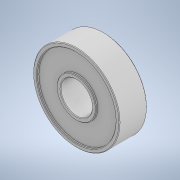
# Autodesk Inventor part: SS608-2RS
Saved by Autodesk Inventor 2021 (Build 250183000, 183)
## iProperties
Created: 2021-02-26
Part Number: SS608-2RS
Material: Generic
Document SubType Name: Modeling
Designer: Viktor
Density: 1 g/cm^3
Appearance: Default
Author: Viktor
Autodesk Inventor part; units mm, degrees
ref_plane "YZ Plane" through (0, 0, 0) normal (1, 0, 0) x (0, 1, 0)
ref_plane "XZ Plane" through (0, 0, 0) normal (0, 1, 0) x (-1, 0, 0)
ref_plane "XY Plane" through (0, 0, 0) normal (0, 0, 1) x (1, 0, 0)
sketch "Sketch1" plane through (0, 0, 0) normal (0, 0, 1) x (1, 0, 0)
  circle A0 centre (0, 0) radius 11
  circle A1 centre (0, 0) radius 4
  dimension "d0" = 22
  dimension "d1" = 8
  constraints: 2 centre point, 2 coincident
  measures "d0" diameter of A0
  measures "d1" diameter of A1
extrude "Extrusion1" add sketch "Sketch1" along normal mid plane 7
sketch "Sketch2" plane through (0, 0, 3.5) normal (0, 0, 1) x (1, 0, 0)
  circle A0 centre (0, 0) radius 10
  circle A1 centre (0, 0) radius 5
  circle A2 centre (0, 0) radius 11 projected
  circle A3 centre (0, 0) radius 4 projected
  dimension "d4" = 1
  dimension "d5" = 1
  constraints: 2 centre point, 2 coincident
  measures "d4" radial gap between concentric circles of A2 A0
  measures "d5" radial gap between concentric circles of A3 A1
extrude "Extrusion2" cut sketch "Sketch2" against normal blind 0.5 contours A0
mirror "Mirror1" about plane through (0, 0, 0) normal (0, 0, 1) of "Extrusion2"
chamfer "Chamfer1" distance 0.15 angle 45 8 edges at (-11, 0, 3.5) (-11, 0, -3.5) (-10, 0, 3.5) (-5, 0, 3.5) (-4, 0, 3.5) (-10, 0, -3.5) (-5, 0, -3.5) (-4, 0, -3.5)
body "Solid1"
